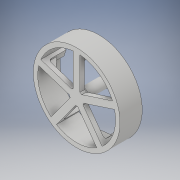
# Autodesk Inventor part: Wheel
Saved by Autodesk Inventor 2019 (Build 230136000, 136)
## iProperties
Created: 2019-02-26
Part Number: Wheel
Material: Generic
Document SubType Name: Modeling
Designer: alarr
Density: 1 g/cm^3
Appearance: Default
Author: alarr
## iProperties of the stored document Wheel_3DPrint.ipt
Created: 2019-02-28
Part Number: Wheel_3DPrint
Material: Generic
Document SubType Name: Modeling
Designer: alarr
Density: 1 g/cm^3
Appearance: Default
Author: alarr
Autodesk Inventor part; units mm, degrees
ref_plane "YZ Plane" through (0, 0, 0) normal (1, 0, 0) x (0, 1, 0)
ref_plane "XZ Plane" through (0, 0, 0) normal (0, 1, 0) x (-1, 0, 0)
ref_plane "XY Plane" through (0, 0, 0) normal (0, 0, 1) x (1, 0, 0)
sketch "Sketch1" plane through (0, 0, 0) normal (0, 0, 1) x (1, 0, 0)
  circle A0 centre (0, 0) radius 49.53
  dimension "d0" = 99.06
  constraints: 1 centre point, 1 coincident
  measures "d0" diameter of A0
extrude "Extrusion1" add sketch "Sketch1" along normal blind 25.4
sketch "Sketch2" plane through (0, 0, 0) normal (0, 0, -1) x (-1, 0, 0)
  circle A0 centre (0, 0) radius 49.53 projected
  circle A1 centre (0, 0) radius 40.64
  circle A2 centre (0, 0) radius 5.715
  dimension "d3" = 8.89
  dimension "d4" = 11.43
  constraints: 2 centre point, 2 coincident
  measures "d4" diameter of A2
extrude "Extrusion2" cut sketch "Sketch2" against normal blind 20.32 contours A1
sketch "Sketch3" plane through (0, 0, 0) normal (0, 0, -1) x (-1, 0, 0)
  circle A0 centre (0, 0) radius 5.715 projected
  circle A1 centre (0, 0) radius 5.715
  constraints: 1 centre point, 1 coincident, 1 concentric
extrude "Extrusion3" add sketch "Sketch3" along normal blind 5.08
sketch "Sketch4" plane through (0, 0, -5.08) normal (0, 0, -1) x (-1, 0, 0)
  circle A0 centre (0, 0) radius 5.715
  circle A1 centre (0, 0) radius 2.54 construction
  line L0 (1.778, 1.813923) -> (1.778, -1.813923)
  line L1 (0, 0) -> (0, 2.54) construction
  line L2 (-1.778, 1.813923) -> (-1.778, -1.813923)
  arc A2 (1.778, 1.813923) -> (-1.778, 1.813923) centre (0, 0) ccw
  arc A3 (-1.778, -1.813923) -> (1.778, -1.813923) centre (0, 0) ccw
  dimension "d9" = 5.08
  dimension "d10" = 3.556
  constraints: 8 point on circle, 6 end point, 3 centre point, 2 symmetric about line, 2 vertical, 1 coincident, 1 concentric
  measures "d9" diameter of A1
  measures "d10" distance between parallel lines of L0 L2
extrude "Extrusion4" cut sketch "Sketch4" against normal blind 7.62 contours L0 A3 L2 A2
sketch "Sketch5" plane through (0, 0, 25.4) normal (0, 0, 1) x (1, 0, 0)
  circle A0 centre (0, 0) radius 5.715
  circle A1 centre (0, 0) radius 49.53
  circle A2 centre (0, 0) radius 8.255 construction
  circle A3 centre (0, 0) radius 44.45 construction
  line L0 (-3.81, 7.323177) -> (-3.81, 44.286413)
  line L1 (0, 0) -> (0, 44.45) construction
  line L2 (3.81, 7.323177) -> (3.81, 44.286413)
  line L3 (-8.14211, -1.360539) -> (-43.296237, 10.061729)
  line L4 (-5.787401, 5.886512) -> (-40.941527, 17.30878)
  line L5 (-1.222101, -8.164037) -> (-22.948546, -38.067923)
  line L6 (-7.38681, -3.685113) -> (-29.113255, -33.588999)
  line L7 (7.38681, -3.685113) -> (29.113255, -33.588999)
  line L8 (1.222101, -8.164037) -> (22.948546, -38.067923)
  line L9 (5.787401, 5.886512) -> (40.941527, 17.30878)
  line L10 (8.14211, -1.360539) -> (43.296237, 10.061729)
  arc A4 (-3.81, 44.286413) -> (-40.941527, 17.30878) centre (0, 0) ccw
  arc A5 (-3.81, 7.323177) -> (-5.787401, 5.886512) centre (0, 0) ccw
  arc A6 (7.38681, -3.685113) -> (8.14211, -1.360539) centre (0, 0) ccw
  arc A7 (-1.222101, -8.164037) -> (1.222101, -8.164037) centre (0, 0) ccw
  arc A8 (-8.14211, -1.360539) -> (-7.38681, -3.685113) centre (0, 0) ccw
  arc A9 (-43.296237, 10.061729) -> (-29.113255, -33.588999) centre (0, 0) ccw
  arc A10 (-22.948546, -38.067923) -> (22.948546, -38.067923) centre (0, 0) ccw
  arc A11 (29.113255, -33.588999) -> (43.296237, 10.061729) centre (0, 0) ccw
  arc A12 (40.941527, 17.30878) -> (3.81, 44.286413) centre (0, 0) ccw
  arc A13 (5.787401, 5.886512) -> (3.81, 7.323177) centre (0, 0) ccw
  dimension "d13" = 2.54
  dimension "d14" = 5.08
  dimension "d16" = 7.62
  dimension "d19" = 360
  constraints: 22 end point, 22 point on circle, 11 centre point, 5 concentric, 2 symmetric about line, 2 vertical, 1 coincident, 39 other
  measures "d16" distance between parallel lines of L2 L0
extrude "Extrusion5" cut sketch "Sketch5" against normal blind 25.4 contours A5 L4 A4 L0 | L2 A12 L9 A13 | A8 L6 A9 L3 | A7 L8 A10 L5 | A6 L10 A11 L7
sketch "Sketch8" plane through (0, 0, 0) normal (1, 0, 0) x (0, 1, 0)
  line L0 (40.64, 10.16) -> (30.48, 20.32)
  line L1 (40.64, 10.16) -> (40.64, 0) construction
  line L2 (40.64, 0) -> (40.64, 20.32) construction
  line L3 (40.64, 10.16) -> (40.64, 20.32)
  line L4 (40.64, 20.32) -> (40.461012, 20.32)
  line L5 (7.323177, 20.32) -> (40.461012, 20.32) construction
  line L6 (30.48, 20.32) -> (40.64, 20.32)
  point P0 (0, 0)
  constraints: 8 end point, 2 equal length, 1 collinear, 1 midpoint, 1 point on line
extrude "Rib1" add sketch "Sketch8" along normal mid plane 2.54 rib yes fills toward (35.595355, 15.275355) open curves L0
pattern_circular "Circular Pattern1" count 5 over 360 about axis through (0, 0, 0) along (0, 0, 1) of "Rib1"
fillet "Fillet1" radius 3.175 1 edges at (5.715, 0, 20.32)
fillet "Fillet2" radius 3.175 10 edges at (-25.8968, -31.3204, 20.32) (-21.7849, -34.3078, 20.32) (21.7849, -34.3078, 20.32) (25.8968, -31.3204, 20.32) (-39.3606, 10.117, 20.32) (-37.79, 14.9507, 20.32) (-2.5412, 40.5605, 20.32) (2.5412, 40.5605, 20.32) (39.3606, 10.117, 20.32) (37.79, 14.9507, 20.32)
body "Solid1"
